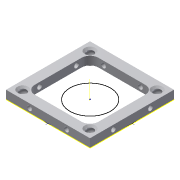
# Autodesk Inventor part: 10_Base_v2
Saved by Autodesk Inventor 2019 (Build 230136000, 136)
## iProperties
Created: 2017-06-20
Part Number: 10_Base_v2
Material: Generisch
Document SubType Name: Modeling
Designer: diederichbenedict
Density: 1 g/cm^3
Appearance: Weiß
Mass: 7.87446 g
Surface Area: 71.4468 cm^2
Volume: 7.87446 cm^3
d_part: 50,000 mm
d_o: 40,000 mm
d_i: 40,000 mm
Author: diederichbenedict
Autodesk Inventor part; units mm, degrees
ref_plane "YZ Plane" through (0, 0, 0) normal (1, 0, 0) x (0, 1, 0)
ref_plane "XZ Plane" through (0, 0, 0) normal (0, 1, 0) x (-1, 0, 0)
sketch "Skizze1" plane through (0, 0, 0) normal (0, 0, 1) x (1, 0, 0)
  line L0 (-25, 25) -> (25, 25)
  line L1 (25, 25) -> (25, -25)
  line L2 (25, -25) -> (-25, -25)
  line L3 (-25, -25) -> (-25, 25)
  line L4 (-25, 25) -> (25, -25) construction
  line L5 (25, 25) -> (-25, -25) construction
  line L6 (20, 20) -> (23, 20) construction
  line L7 (-20, -20) -> (20, -20) construction
  line L8 (20, -20) -> (20, 20) construction
  line L9 (20, 20) -> (-20, 20) construction
  line L10 (-20, 20) -> (-20, -20) construction
  line L11 (-20, -20) -> (20, 20) construction
  line L12 (20, -20) -> (-20, 20) construction
  line L13 (-14, 19) -> (14, 19)
  line L14 (19, 14) -> (19, -14)
  line L15 (14, -19) -> (-14, -19)
  line L16 (-19, -14) -> (-19, 14)
  line L17 (-19, 19) -> (19, -19) construction
  line L18 (19, 19) -> (-19, -19) construction
  arc A0 (14, -19) -> (19, -14) centre (14, -14) ccw
  arc A1 (19, 14) -> (14, 19) centre (14, 14) ccw
  arc A2 (-14, 19) -> (-19, 14) centre (-14, 14) ccw
  arc A3 (-19, -14) -> (-14, -19) centre (-14, -14) ccw
  point P0 (0, 0)
  point P1 (0, 0)
  dimension "d2" = 50
  dimension "d3" = 50
  dimension "d273" = 40
  dimension "d274" = 40
  dimension "d275" = 38
  dimension "d276" = 38
  dimension "d277" = 5
  constraints: 38 end point, 8 point on circle, 8 point on line, 8 tangent, 6 midpoint, 6 parallel, 4 centre point, 4 horizontal, 3 equal radius, 3 perpendicular
  measures "d2" distance of L1.end L2.end
  measures "d3" distance of L0.end L1.end
  measures "d273" distance of L9.end L6.start
  measures "d274" distance of L6.start L7.end
  measures "d275" distance of L17.end L18.end
  measures "d276" distance of L18.start L17.end
  measures "d277" radius of A0
extrude "Extrusion1" add sketch "Skizze1" along normal blind 5
ref_plane "Arbeitsebene1" through (-25, -20, 0) normal (0, -1, 0) x (1, 0, 0)
sketch "Skizze5" plane through (-25, -20, 0) normal (0, -1, 0) x (1, 0, 0)
  line L0 (50, 0) -> (0, 0) projected
  line L1 (0, 0) -> (0, 5) projected
  line L2 (5, -0.15) -> (5, 5.15)
  line L3 (5, 1) -> (7.1846, 1)
  line L4 (2.7, -1.6033) -> (2.7, 1.1838)
  line L5 (5, -1.6033) -> (5, -0.15)
  arc A0 (2.7, 3.8162) -> (4.1211, 0) centre (5, 2.5) ccw
  arc A1 (5, -0.15) -> (5, 5.15) centre (5, 2.5) ccw
  line L6 (7.1846, 1) -> (8.3346, -0.15)
  line L7 (8.3346, -0.15) -> (5, -0.15)
  line L8 (5, 2.5) -> (6.8859, 2.5)
  line L9 (7.1846, 4) -> (8.3346, 5.15)
  line L10 (8.3346, 5.15) -> (5, 5.15)
  point P0 (25, 0)
  point P1 (40, 8)
  point P2 (6.6949, -37.8745)
  dimension "d237" = 2.5
  dimension "d238" = 5
  dimension "d240" = 2.3
  dimension "d247" = 135
  dimension "d248" = 1.5
  dimension "d249" = 2.65
  constraints: 18 end point, 7 point on circle, 3 point on line, 2 centre point, 2 horizontal, 2 perpendicular, 1 parallel
  measures "d237" distance from line of L8.start L0
  measures "d238" distance from line of L1 L8.start
  measures "d240" distance between parallel lines of L4 L2
  measures "d247" angle of L7 L6
  measures "d248" distance from line of L8.start L3
  measures "d249" radius of A1
revolve "Umdrehung1" cut sketch "Skizze5" angle 360 about axis through (-20, -20, -0.15) along (0, 0, 1) contours L6 L7 A1 L0 | L0 A1 L6 | A1 L2 L0 | L0 L2 L3 A1 | L3 L2 A1 | A1 L10 L9
pattern_linear "Rechteckige Anordnung7" count 2 spacing 40 along (1, 0, 0) count 2 spacing 40 along (0, 1, 0) of "Umdrehung1"
sketch "Skizze16" plane through (0, 0, 0) normal (0, 0, -1) x (-1, 0, 0)
  line L0 (25, 25) -> (-25, 25) projected
  line L1 (-25, 25) -> (-25, -25) projected
  line L2 (-25, -25) -> (25, -25) projected
  line L3 (25, -25) -> (25, 25) projected
  circle A0 centre (0, 0) radius 25
  line L4 (-25, -25) -> (25, -25) projected
  line L5 (25, 25) -> (-25, 25) projected
  line L6 (25, 25) -> (25, -25) projected
  circle A1 centre (-20, 20) radius 3.1846 projected
  circle A2 centre (20, 20) radius 3.1846 projected
  circle A3 centre (20, -20) radius 3.1846 projected
  circle A4 centre (-20, -20) radius 3.1846 projected
  point P0 (0, -25)
  point P1 (-25, 0)
  point P2 (0, 25)
  point P3 (25, 0)
  constraints: 4 midpoint, 1 coincident, 1 horizontal alignment, 2 other
sketch "Skizze17" plane through (25, -15.5, 1) normal (-1, 0, 0) x (0, 0, 1)
  line L0 (-1, 40.5) -> (-1, -9.5) projected
  line L1 (-1, 40.5) -> (4, 40.5) projected
  line L2 (4, -9.5) -> (4, 40.5) projected
  line L3 (4, -9.5) -> (4, 40.5) projected
  line L4 (-1, -9.5) -> (4, -9.5) projected
  line L5 (-1, 40.5) -> (-1, -9.5) projected
  circle A0 centre (1.5, 26.5) radius 1.4
  circle A1 centre (1.5, 4.5) radius 1.4
  line L6 (-1, 40.5) -> (4, 40.5) projected
  line L7 (-1, -9.5) -> (4, -9.5) projected
  dimension "d241" = 2.8
  dimension "d242" = 2.8
  dimension "d243" = 14
  dimension "d1" = 14
  dimension "d253" = 2.5
  dimension "d254" = 2.5
  constraints: 2 centre point
  measures "d241" diameter of A0
  measures "d242" diameter of A1
  measures "d243" distance from line of A0.centre L1
  measures "d1" distance from line of A1.centre L4
  measures "d253" distance from line of A1.centre L3
  measures "d254" distance from line of A0.centre L2
extrude "Extrusion12" cut sketch "Skizze17" along normal blind 10 contours A0 | A1
sketch "Sketch24" plane through (0, 0, 0) normal (0, 0, -1) x (-1, 0, 0)
  circle A0 centre (20, -20) radius 3.1846 projected
  circle A1 centre (-20, -20) radius 3.1846 projected
  circle A2 centre (20, 20) radius 3.1846 projected
  circle A3 centre (-20, 20) radius 3.1846 projected
  line L0 (25, 25) -> (-25, 25) projected
  line L1 (-25, 25) -> (-25, -25) projected
  line L2 (-25, -25) -> (25, -25) projected
  line L3 (25, -25) -> (25, 25) projected
  circle A4 centre (0, 0) radius 12.0567
  constraints: 1 centre point, 1 coincident
pattern_circular "Circular Pattern4" count 4 over 360 about axis through (0, 0, 0) along (0, 0, 1) of "Extrusion12"
equation "\"d2\" = d_part"
equation "\"d3\" = d_part"
equation "\"d_i\" = 40"
equation "\"d_o\" = 40"
equation "\"d_part\" = 50"
equation "\"d6\" = 0"
equation "\"d7\" = 0"
equation "\"d8\" = 0"
equation "\"d9\" = 0"
equation "\"d13\" = 0"
equation "\"d14\" = 0"
equation "\"d20\" = 0"
equation "\"d21\" = 0"
equation "\"d22\" = 0"
equation "\"d23\" = 0"
equation "\"d24\" = 0"
equation "\"d25\" = 3"
equation "\"d26\" = 0"
equation "\"d27\" = 0"
equation "\"d28\" = 0"
equation "\"d29\" = 0"
equation "\"d30\" = 0"
equation "\"d31\" = 0"
equation "\"d32\" = 0"
equation "\"d33\" = 0"
equation "\"d34\" = 0"
equation "\"d46\" = 0"
equation "\"d47\" = 0"
equation "\"d48\" = 0"
equation "\"d50\" = 0"
equation "\"d51\" = 0"
equation "\"d52\" = 0"
equation "\"d53\" = 0"
equation "\"d54\" = 0"
equation "\"d55\" = 0"
equation "\"d56\" = 0"
equation "\"d57\" = 0"
equation "\"d58\" = 0"
equation "\"d59\" = 0"
